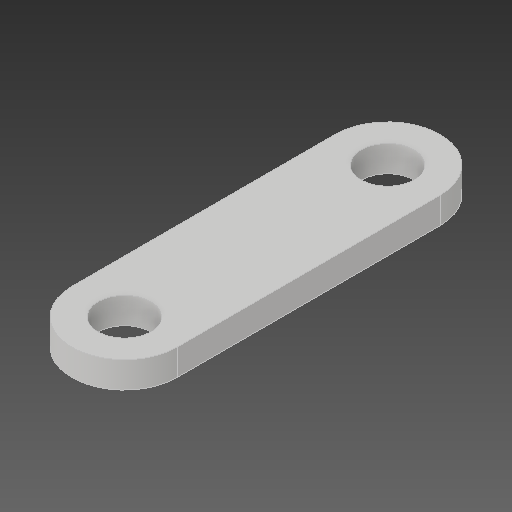
# Autodesk Inventor part: penompang capit
Saved by Autodesk Inventor 2019 (Build 230136000, 136)
## iProperties
Created: 2016-12-01
Part Number: penompang capit
Material: Generic
Document SubType Name: Modeling
Designer: MuhammadArdian
Density: 1 g/cm^3
Appearance: Default
Author: MuhammadArdian
Autodesk Inventor part; units mm, degrees
ref_plane "YZ Plane" through (0, 0, 0) normal (1, 0, 0) x (0, 1, 0)
ref_plane "XZ Plane" through (0, 0, 0) normal (0, 1, 0) x (-1, 0, 0)
ref_plane "XY Plane" through (0, 0, 0) normal (0, 0, 1) x (1, 0, 0)
sketch "Sketch1" plane through (0, 0, 0) normal (0, 1, 0) x (-1, 0, 0)
  arc A0 (10, 25) -> (-10, 25) centre (0, 25) ccw
  arc A1 (-10, -25) -> (10, -25) centre (0, -25) ccw
  circle A2 centre (0, 25) radius 5
  circle A3 centre (0, -25) radius 5
  line L0 (10, 25) -> (10, -25)
  line L1 (-10, 25) -> (-10, -25)
  point P0 (0, 0)
  dimension "d8" = 10
  dimension "d9" = 50
  dimension "d10" = 50
  constraints: 4 centre point, 4 end point, 4 point on circle, 2 coincident, 2 tangent
  measures "d8" diameter of A2
  measures "d9" distance of L0.start L0.end
  measures "d10" distance of L1.start L1.end
extrude "Extrusion1" add sketch "Sketch1" along normal blind 5
body "Solid1"
